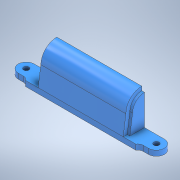
# Autodesk Inventor part: battery mount rear
Saved by Autodesk Inventor 2022 (Build 260153000, 153)
## iProperties
Created: 2023-01-31
Part Number: battery mount rear
Material: Generic
Document SubType Name: Modeling
Designer: scott
Density: 1 g/cm^3
Appearance: Default
Author: scott
Autodesk Inventor part; units mm, degrees
ref_plane "YZ Plane" through (0, 0, 0) normal (1, 0, 0) x (0, 1, 0)
ref_plane "XZ Plane" through (0, 0, 0) normal (0, 1, 0) x (-1, 0, 0)
ref_plane "XY Plane" through (0, 0, 0) normal (0, 0, 1) x (1, 0, 0)
sketch "Sketch1" plane through (0, 0, 0) normal (0, 1, 0) x (-1, 0, 0)
  line L0 (0, 0) -> (24.5, 0)
  line L1 (24.5, 0) -> (24.5, 5)
  line L2 (24.5, 5) -> (0, 5)
  line L3 (0, 5) -> (0, 0)
  circle A0 centre (24.5, 2) radius 3
  circle A1 centre (24.5, 2) radius 1
  line L4 (0, 0) -> (15.5, 0)
  line L5 (15.5, 0) -> (15.5, 3)
  line L6 (15.5, 3) -> (0, 3)
  line L7 (0, 3) -> (0, 0)
  line L8 (0, 3) -> (6.5, 3)
  line L9 (6.5, 3) -> (6.5, 6)
  line L10 (6.5, 6) -> (0, 6)
  line L11 (0, 6) -> (0, 3)
  line L12 (6.5, 6) -> (20.5, 6)
  line L13 (20.5, 6) -> (20.5, 5)
  line L14 (20.5, 5) -> (6.5, 5)
  line L15 (6.5, 5) -> (6.5, 6)
  circle A2 centre (22.5, 7) radius 2
  line L16 (20.5, 6) -> (24.5, 6)
  line L17 (24.5, 6) -> (24.5, 5)
  line L18 (24.5, 5) -> (20.5, 5)
  line L19 (20.5, 5) -> (20.5, 6)
  line L20 (15.5, 0) -> (24.5, 0)
  line L21 (24.5, 0) -> (24.5, -1)
  line L22 (24.5, -1) -> (15.5, -1)
  line L23 (15.5, -1) -> (15.5, 0)
  point P0 (22.5, 5)
  point P1 (20.7679, 6)
  point P2 (0, 3)
  point P3 (22.2639, 0)
  point P4 (0, 5)
  dimension "d1" = 6
  dimension "d0" = 24.5
  dimension "d2" = 2
  dimension "d3" = 2
  dimension "d4" = 3
  dimension "d5" = 3
  dimension "d6" = 9
  dimension "d7" = 3
  dimension "d8" = 18
  dimension "d9" = 4
  dimension "d10" = 4
  dimension "d11" = 2
  constraints: 48 end point, 12 parallel, 6 horizontal, 6 perpendicular, 2 centre point, 2 point on line, 1 coincident, 1 tangent, 3 other
  measures "d0" distance of L0.start L0.end
  measures "d2" diameter of A1
  measures "d3" distance from line of L0 point (24.5, 2)
  measures "d4" distance from line of point (24.5, 2) L2
  measures "d5" distance between parallel lines of L0 L6
  measures "d6" distance from line of point (24.5, 2) L5
  measures "d7" distance between parallel lines of L8 L10
  measures "d8" distance from line of point (24.5, 2) L9
  measures "d9" distance from line of L13 point (24.5, 2)
  measures "d10" diameter of A2
  measures "d11" distance from line of L13 A2.centre
extrude "Extrusion1" add sketch "Sketch1" along normal blind 2 contours L5 L6 L9 L2 A0 L0 | L0 A0 L22 L23 | L3 L2 L9 L6 | A0 L1 A1 L0 | L0 L21 A0 | L11 L10 L9 L2 | L1 A1 A0 L21 | L9 L12 L13 L2 | L2 L13 L16 A2
sketch "Sketch2" plane through (0, 0, 6) normal (1, 0, 0) x (0, 0, -1)
  line L0 (0, 0) -> (0, 2) projected
  line L1 (0, 2) -> (3, 2)
  line L2 (3, 2) -> (3, 12)
  line L3 (3, 12) -> (0, 12)
  line L4 (0, 12) -> (0, 2)
  line L5 (3, 0) -> (3, 2) projected
  line L6 (0, 12) -> (7, 12)
  line L7 (7, 12) -> (7, 15)
  line L8 (7, 15) -> (0, 15)
  line L9 (0, 15) -> (0, 12)
  circle A0 centre (7, 9) radius 3
  line L10 (4, 9) -> (4, 0)
  line L11 (3, 0) -> (5, 0) projected
  line L12 (3, 0) -> (3, 12)
  circle A1 centre (7, 9) radius 6
  line L13 (0, 2) -> (1, 2) projected
  line L14 (0, 2) -> (1, 9)
  point P0 (6, 0)
  point P1 (3, 9)
  point P2 (4, 6.7639)
  dimension "d20" = 6
  dimension "d14" = 10
  dimension "d15" = 0
  dimension "d16" = 7
  dimension "d17" = 3
  dimension "d21" = 3
  dimension "d22" = 7
  constraints: 22 end point, 5 parallel, 2 horizontal, 2 perpendicular, 2 point on circle, 1 centre point, 1 coincident, 1 midpoint, 3 other
  measures "d14" distance of L2.end L1.end
  measures "d15" distance between parallel lines of L2 L5
  measures "d16" distance of L8.end L7.end
  measures "d17" distance of L7.end L6.end
  measures "d21" distance from line of point (7, 9) L6
  measures "d22" distance from line of L4 point (7, 9)
extrude "Extrusion2" add sketch "Sketch2" against normal blind 16 contours L14 A1 L2 L1 | A1 L3 L2 | L2 A1 L10 L11 L5 | A1 L7 L6 L3 | L2 L6 A0 L10 A1
sketch "Sketch3" plane through (-16, 0, 6) normal (-1, 0, 0) x (0, 0, 1)
  arc A0 (-4, 9) -> (-7, 12) centre (-7, 9) ccw projected
  circle A1 centre (-7, 9) radius 2
  line L0 (-7, 12) -> (-7, 9)
  line L1 (-7, 9) -> (-7, 0)
  line L2 (-7, 0) -> (-7, 2) projected
  circle A2 centre (-7, 9) radius 6
  line L3 (-7, 15) -> (-7, 9)
  arc A3 (-1, 9) -> (-7, 15) centre (-7, 9) ccw projected
  line L4 (0, 2) -> (-1, 9) projected
  line L5 (-1, 9) -> (0, 2)
  line L6 (-1, 2) -> (-7, 2) projected
  line L7 (0, 2) -> (-7, 2)
  circle A4 centre (-7, 9) radius 4.5
  line L8 (-2.5, 9) -> (-1, 9)
  line L9 (-1, 2) -> (0, 2) projected
  line L10 (0, 2) -> (-1.5, 2)
  line L11 (-1.5, 2) -> (-2.5, 9)
  point P0 (-6, 0)
  point P1 (-6, 2)
  point P2 (-7, 13.5)
  point P3 (-7, 12)
  point P4 (-1.5, 2)
  dimension "d23" = 4
  dimension "d24" = 9
  dimension "d25" = 1.5
  constraints: 16 end point, 3 centre point, 3 coincident, 3 collinear, 3 point on circle, 2 point on line, 1 horizontal, 1 vertical
  measures "d23" diameter of A1
  measures "d24" diameter of A4
  measures "d25" distance of L4.start L10.end
extrude "Extrusion3" add sketch "Sketch3" along normal blind 1 and the other way blind 1 contours A1 L1 L0 | A1 L0 L3 A4 L1 | A4 L11 A2 L1 | A2 L11 L6 L1 picked at (-5.7494, 8.5624) picked at (-6.0599, 11.9521)
sketch "Sketch4" plane through (-15.5, 0, -1) normal (0, 0, -1) x (-1, 0, 0)
  line L0 (-0.5, 2) -> (-0.5, 9) projected
  line L1 (0, 0) -> (0, 2) projected
  line L2 (-0.5, 2) -> (0, 2)
  line L3 (0, 2) -> (0, 0)
  line L4 (0, 0) -> (-0.5, 0)
  line L5 (-0.5, 0) -> (-0.5, 2)
  point P0 (-15.5, 0)
  constraints: 8 end point, 2 parallel, 1 horizontal, 1 perpendicular
extrude "Extrusion4" add sketch "Sketch4" against normal up to surface (3 mm away)
mirror "Mirror1" about plane through (0, 0, 6) normal (1, 0, 0) of "Extrusion1", "Extrusion2", "Extrusion3", "Extrusion4"
body "Solid1"
